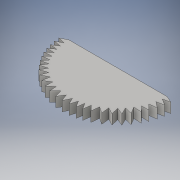
# Autodesk Inventor part: Part4
Saved by Autodesk Inventor 2016 (Build 200138000, 138)
## iProperties
Created: 2016-11-13
Part Number: Part4
Material: Generic
Document SubType Name: Modeling
Designer: adam fishburn
Density: 1 g/cm^3
Appearance: Default
Author: adam fishburn
Autodesk Inventor part; units mm, degrees
ref_plane "YZ Plane" through (0, 0, 0) normal (1, 0, 0) x (0, 1, 0)
ref_plane "XZ Plane" through (0, 0, 0) normal (0, 1, 0) x (-1, 0, 0)
ref_plane "XY Plane" through (0, 0, 0) normal (0, 0, 1) x (1, 0, 0)
sketch "Sketch1" plane through (0, 0, 0) normal (0, 1, 0) x (-1, 0, 0)
  line L0 (0, 0) -> (101.6, 0)
  line L1 (101.6, 0) -> (101.6, -101.6)
  line L2 (101.6, -101.6) -> (0, -101.6)
  line L3 (0, -101.6) -> (0, 0)
  dimension "d0" = 101.6
  dimension "d1" = 101.6
  constraints: 8 end point, 2 parallel, 1 horizontal, 1 perpendicular
  measures "d0" distance of L1.end L2.end
  measures "d1" distance of L0.end L1.end
extrude "Extrusion1" add sketch "Sketch1" along normal blind 6.35 draft 0.25
sketch "Sketch2" plane through (0, 6.35, 0) normal (0, 1, 0) x (1, 0, 0)
  line L0 (-82.5492, 50.8025) -> (-86.8726, 48.5826)
  line L1 (-86.8726, 48.5826) -> (-82.3808, 47.537)
  line L2 (-82.3808, 47.537) -> (-86.5353, 45.4037)
  line L3 (-86.5353, 45.4037) -> (-81.9297, 44.5615)
  line L4 (-81.9297, 44.5615) -> (-85.8551, 42.0104)
  line L5 (-85.8551, 42.0104) -> (-81.2075, 41.6704)
  line L6 (-81.2075, 41.6704) -> (-84.931, 38.9182)
  line L7 (-84.931, 38.9182) -> (-80.2411, 38.9182)
  line L8 (-80.2411, 38.9182) -> (-83.7111, 35.8686)
  line L9 (-83.7111, 35.8686) -> (-78.9909, 36.1982)
  line L10 (-78.9909, 36.1982) -> (-82.2207, 32.9446)
  line L11 (-82.2207, 32.9446) -> (-77.3914, 33.4556)
  line L12 (-77.3914, 33.4556) -> (-80.2618, 29.8701)
  line L13 (-80.2618, 29.8701) -> (-75.5543, 30.9218)
  line L14 (-75.5543, 30.9218) -> (-78.0086, 27.0147)
  line L15 (-78.0086, 27.0147) -> (-73.2491, 28.3512)
  line L16 (-75.4686, 24.3897) -> (-70.7203, 26.0798)
  line L17 (-70.7203, 26.0798) -> (-72.3407, 21.7822)
  line L18 (-72.3407, 21.7822) -> (-67.7356, 23.947)
  line L19 (-67.7356, 23.947) -> (-68.5334, 19.3111)
  line L20 (-68.5334, 19.3111) -> (-64.1946, 22.0167)
  line L21 (-64.1946, 22.0167) -> (-64.3717, 17.3062)
  line L22 (-64.3717, 17.3062) -> (-60.4516, 20.5554)
  line L23 (-60.4516, 20.5554) -> (-60.1774, 15.8989)
  line L24 (-60.1774, 15.8989) -> (-56.5068, 19.5698)
  line L25 (-56.5068, 19.5698) -> (-55.1527, 14.9241)
  line L26 (-55.1527, 14.9241) -> (-52.5263, 19.0996)
  line L27 (-52.5263, 19.0996) -> (-50.7684, 14.6609)
  line L28 (-50.7684, 14.6609) -> (-48.585, 19.1298)
  line L29 (-48.585, 19.1298) -> (-46.5035, 14.9171)
  line L30 (-46.5035, 14.9171) -> (-45.1599, 19.5574)
  line L31 (-45.1599, 19.5574) -> (-42.5914, 15.6053)
  line L32 (-42.5914, 15.6053) -> (-41.7527, 20.3686)
  line L33 (-41.7527, 20.3686) -> (-39.298, 16.5397)
  line L34 (-39.298, 16.5397) -> (-38.6769, 21.4578)
  line L35 (-38.6769, 21.4578) -> (-35.49, 18.0635)
  line L36 (-35.49, 18.0635) -> (-35.1146, 23.1972)
  line L37 (-35.1146, 23.1972) -> (-30.9781, 20.581)
  line L38 (-30.9781, 20.581) -> (-31.5036, 25.5886)
  line L39 (-31.5036, 25.5886) -> (-27.2251, 23.4077)
  line L40 (-27.2251, 23.4077) -> (-28.4283, 28.2724)
  line L41 (-28.4283, 28.2724) -> (-23.9858, 26.5691)
  line L42 (-23.9858, 26.5691) -> (-26.0364, 30.9313)
  line L43 (-26.0364, 30.9313) -> (-21.3587, 29.8388)
  line L44 (-21.3587, 29.8388) -> (-23.7723, 34.1409)
  line L45 (-23.7723, 34.1409) -> (-18.848, 33.9105)
  line L46 (-18.848, 33.9105) -> (-22.0511, 37.3262)
  line L47 (-22.0511, 37.3262) -> (-17.264, 37.3262)
  line L48 (-17.264, 37.3262) -> (-20.7009, 40.6952)
  line L49 (-20.7009, 40.6952) -> (-15.918, 41.3408)
  line L50 (-15.918, 41.3408) -> (-19.7237, 44.293)
  line L51 (-19.7237, 44.293) -> (-15.0837, 45.2689)
  line L52 (-15.0837, 45.2689) -> (-19.1835, 47.8849)
  line L53 (-19.1835, 47.8849) -> (-14.7085, 48.8843)
  line L54 (-14.7085, 48.8843) -> (-19.0492, 50.8025)
  line L55 (-75.4686, 24.3897) -> (-73.2491, 28.3512)
  circle A0 centre (-50.8, 50.8) radius 31.7508
  circle A1 centre (-50.8, 50.8) radius 37.6285
  line L56 (-101.6277, 101.6277) -> (0.0277, 101.6277) projected
  line L57 (0.0277, 101.6277) -> (0.0277, -0.0277) projected
  line L58 (-101.6277, 101.6277) -> (0.0277, 101.6277)
  line L59 (0.0277, 101.6277) -> (0.0277, -0.0277)
  line L60 (0.0277, -0.0277) -> (-101.6277, -0.0277) projected
  line L61 (0.0277, -0.0277) -> (-101.6277, -0.0277)
  line L62 (-101.6277, -0.0277) -> (-101.6277, 101.6277)
  constraints: 120 end point, 3 horizontal, 3 perpendicular, 1 centre point, 1 coincident, 3 other
extrude "Extrusion2" cut sketch "Sketch2" against normal blind 6.35 contours L56 L57 L60 L62
sketch "Sketch3" plane through (-50.8, 6.35, -50.8) normal (0, 1, 0) x (1, 0, 0)
  line L0 (-31.7492, 0.0025) -> (-36.0726, -2.2174)
  line L1 (-36.0726, -2.2174) -> (-31.5808, -3.263)
  line L2 (-31.5808, -3.263) -> (-35.7353, -5.3963)
  line L3 (-35.7353, -5.3963) -> (-31.1298, -6.2385)
  line L4 (-31.1298, -6.2385) -> (-35.0551, -8.7896)
  line L5 (-35.0551, -8.7896) -> (-30.4075, -9.1296)
  line L6 (-30.4075, -9.1296) -> (-34.131, -11.8818)
  line L7 (-34.131, -11.8818) -> (-29.4411, -11.8818)
  line L8 (-29.4411, -11.8818) -> (-32.9111, -14.9315)
  line L9 (-32.9111, -14.9315) -> (-28.191, -14.6019)
  line L10 (-28.191, -14.6019) -> (-31.4207, -17.8554)
  line L11 (-31.4207, -17.8554) -> (-26.5914, -17.3444)
  line L12 (-26.5914, -17.3444) -> (-29.4619, -20.9299)
  line L13 (-29.4619, -20.9299) -> (-24.7544, -19.8782)
  line L14 (-24.7544, -19.8782) -> (-27.2087, -23.7853)
  line L15 (-27.2087, -23.7853) -> (-22.4492, -22.4488)
  line L16 (-24.6686, -26.4103) -> (-19.9203, -24.7202)
  line L17 (-19.9203, -24.7202) -> (-21.5408, -29.0178)
  line L18 (-21.5408, -29.0178) -> (-16.9357, -26.853)
  line L19 (-16.9357, -26.853) -> (-17.7335, -31.489)
  line L20 (-17.7335, -31.489) -> (-13.3947, -28.7833)
  line L21 (-13.3947, -28.7833) -> (-13.5717, -33.4938)
  line L22 (-13.5717, -33.4938) -> (-9.6516, -30.2447)
  line L23 (-9.6516, -30.2447) -> (-9.3774, -34.9011)
  line L24 (-9.3774, -34.9011) -> (-5.7069, -31.2302)
  line L25 (-5.7069, -31.2302) -> (-4.3528, -35.8759)
  line L26 (-4.3528, -35.8759) -> (-1.7263, -31.7005)
  line L27 (-1.7263, -31.7005) -> (0.0315, -36.1391)
  line L28 (0.0315, -36.1391) -> (2.215, -31.6702)
  line L29 (2.215, -31.6702) -> (4.2964, -35.8829)
  line L30 (4.2964, -35.8829) -> (5.64, -31.2426)
  line L31 (5.64, -31.2426) -> (8.2086, -35.1948)
  line L32 (8.2086, -35.1948) -> (9.0473, -30.4314)
  line L33 (9.0473, -30.4314) -> (11.502, -34.2603)
  line L34 (11.502, -34.2603) -> (12.123, -29.3422)
  line L35 (12.123, -29.3422) -> (15.3099, -32.7365)
  line L36 (15.3099, -32.7365) -> (15.6854, -27.6028)
  line L37 (15.6854, -27.6028) -> (19.8219, -30.219)
  line L38 (19.8219, -30.219) -> (19.2964, -25.2114)
  line L39 (19.2964, -25.2114) -> (23.5749, -27.3924)
  line L40 (23.5749, -27.3924) -> (22.3717, -22.5276)
  line L41 (22.3717, -22.5276) -> (26.8141, -24.2309)
  line L42 (26.8141, -24.2309) -> (24.7636, -19.8687)
  line L43 (24.7636, -19.8687) -> (29.4412, -20.9612)
  line L44 (29.4412, -20.9612) -> (27.0277, -16.6591)
  line L45 (27.0277, -16.6591) -> (31.9519, -16.8895)
  line L46 (31.9519, -16.8895) -> (28.7489, -13.4738)
  line L47 (28.7489, -13.4738) -> (33.5359, -13.4738)
  line L48 (33.5359, -13.4738) -> (30.099, -10.1049)
  line L49 (30.099, -10.1049) -> (34.8819, -9.4592)
  line L50 (34.8819, -9.4592) -> (31.0763, -6.5071)
  line L51 (31.0763, -6.5071) -> (35.7163, -5.5311)
  line L52 (35.7163, -5.5311) -> (31.6164, -2.9151)
  line L53 (31.6164, -2.9151) -> (36.0915, -1.9157)
  line L54 (36.0915, -1.9157) -> (31.7508, 0.0025)
  line L55 (-24.6686, -26.4103) -> (-22.4492, -22.4488)
  line L56 (-31.7492, 0.0025) -> (31.7508, 0.0025)
  circle A0 centre (0.0008, 0.0025) radius 37.6862
  point P0 (50.8, -50.8)
  constraints: 114 end point, 3 horizontal, 1 centre point, 1 midpoint
extrude "Extrusion3" cut sketch "Sketch3" against normal blind 6.35
body "Solid1"
